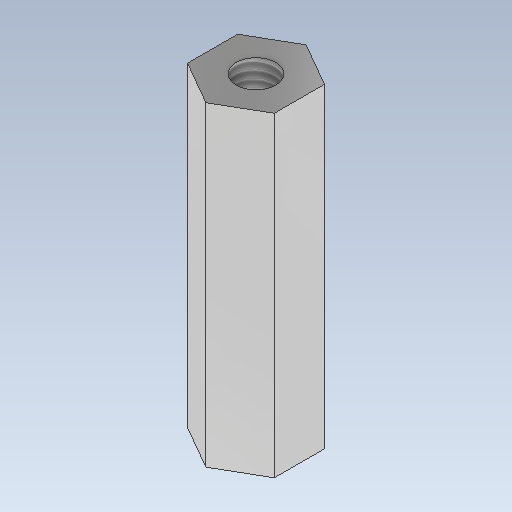
# Autodesk Inventor part: Distance_M3_20
Saved by Autodesk Inventor 2021 (Build 250183000, 183)
## iProperties
Created: 2020-03-25
Part Number: Distance_M3_20
Material: Nickel-Copper Alloy 400
Document SubType Name: Modeling
Designer: ermoz
Density: 8.83 g/cm^3
Appearance: Chrome - Polished
Mass: 5.63933 g
Surface Area: 8.49773 cm^2
Volume: 0.638656 cm^3
Author: ermoz
Autodesk Inventor part; units mm, degrees
ref_plane "YZ Plane" through (0, 0, 0) normal (1, 0, 0) x (0, 1, 0)
ref_plane "XZ Plane" through (0, 0, 0) normal (0, 1, 0) x (-1, 0, 0)
ref_plane "XY Plane" through (0, 0, 0) normal (0, 0, 1) x (1, 0, 0)
sketch "Sketch1" plane through (0, 0, 0) normal (0, 1, 0) x (-1, 0, 0)
  circle A0 centre (0, 0) radius 2.75
  line L0 (2.75, -1.5877) -> (0, -3.1754)
  line L1 (0, -3.1754) -> (-2.75, -1.5877)
  line L2 (-2.75, -1.5877) -> (-2.75, 1.5877)
  line L3 (-2.75, 1.5877) -> (0, 3.1754)
  line L4 (0, 3.1754) -> (2.75, 1.5877)
  line L5 (2.75, 1.5877) -> (2.75, -1.5877)
  circle A1 centre (0, 0) radius 1.25
  point P0 (2.75, 0)
  dimension "d0" = 5.5
  dimension "d1" = 2.5
  constraints: 12 end point, 3 coincident, 1 centre point, 1 horizontal alignment, 1 midpoint, 15 other
  measures "d1" diameter of A1
extrude "Extrusion1" add sketch "Sketch1" along normal blind 30
thread "Thread1" size "M3x0.5" class "6H" standard "ANSI Metric M Profile" full length
sketch "Sketch2" plane through (0, 30, 0) normal (0, 1, 0) x (1, 0, 0)
  line L0 (-7.5964, -8.221) -> (7.9188, -8.221)
  line L1 (7.9188, -8.221) -> (7.9188, 5.8837)
  line L2 (7.9188, 5.8837) -> (-7.5964, 5.8837)
  line L3 (-7.5964, 5.8837) -> (-7.5964, -8.221)
  point P0 (0, 0)
  constraints: 8 end point, 2 parallel, 1 horizontal, 1 perpendicular
extrude "Extrusion2" cut sketch "Sketch2" against normal blind 10
body "Solid1"
